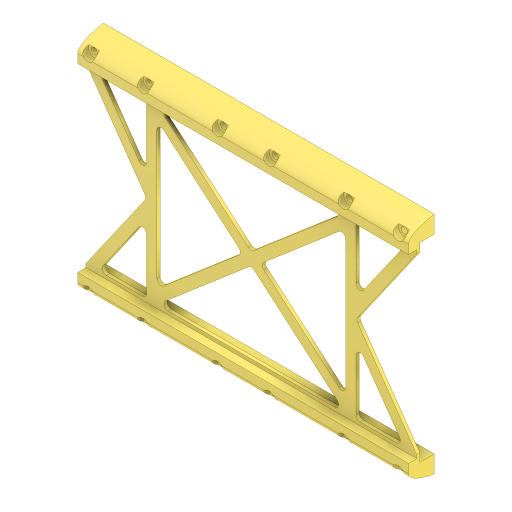
# Autodesk Inventor part: BodyStructure Centre V2
Saved by Autodesk Inventor 2023 (Build 270158000, 158)
## iProperties
Created: 2019-11-07
Part Number: BodyStructure Centre V2
Material: solidworks materials|ABS
Document SubType Name: Modeling
Designer: Jochen
Density: 1.02 g/cm^3
Appearance: 151,157,178
Sending System: SolidWorks 2017
Last Author: Felix
Last Saved: 2021-02-23
Author: Jochen
Autodesk Inventor part; units mm, degrees
ref_plane "YZ Plane" through (0, 0, 0) normal (1, 0, 0) x (0, 1, 0)
ref_plane "XZ Plane" through (0, 0, 0) normal (0, 1, 0) x (-1, 0, 0)
ref_plane "Work Plane1" through (0, 0, 30) normal (0, 0, 1) x (1, 0, 0)
sketch "Sketch1" plane through (0, 0, 30) normal (0, 0, 1) x (1, 0, 0)
  line L0 (-80, -56) -> (80, -56)
  line L1 (80, 56) -> (-80, 56)
  line L2 (80, 42) -> (80, 42)
  line L3 (0, -78.4) -> (0, 78.4) construction
  line L4 (-112, 0) -> (112, 0) construction
  line L5 (-50.6486, -42) -> (-50.6486, -8.7287)
  line L6 (-45.6486, 35.4185) -> (-45.6486, -35.4185)
  line L7 (-50.6486, -8.7287) -> (-73.9, -42)
  line L8 (-80, -42) -> (-50.6486, 0)
  line L9 (50.6486, -8.7287) -> (73.9, -42)
  line L10 (50.6486, -42) -> (50.6486, -8.7287)
  line L11 (45.6486, 35.4185) -> (45.6486, -35.4185)
  line L12 (80, -42) -> (50.6486, 0)
  line L13 (50.6486, 8.7287) -> (73.9, 42)
  line L14 (80, 42) -> (50.6486, 0)
  line L15 (50.6486, 0) -> (50.6486, 0)
  line L16 (50.6486, 8.7287) -> (50.6486, 42)
  line L17 (-50.6486, 0) -> (-50.6486, 0)
  line L18 (-80, 42) -> (-50.6486, 0)
  line L19 (-50.6486, 8.7287) -> (-73.9, 42)
  line L20 (-80, 42) -> (-80, 42)
  line L21 (-50.6486, 8.7287) -> (-50.6486, 42)
  line L22 (73.9, 42) -> (50.6486, 42)
  line L23 (-73.9, 42) -> (-50.6486, 42)
  line L24 (-45.6486, 42) -> (45.6486, 42)
  line L25 (-80, -42) -> (-80, -42)
  line L26 (-50.6486, -42) -> (-73.9, -42)
  line L27 (45.6486, -42) -> (-45.6486, -42)
  line L28 (80, -42) -> (80, -42)
  line L29 (73.9, -42) -> (50.6486, -42)
  line L30 (80, -56) -> (80, -42)
  line L31 (80, 42) -> (80, 56)
  line L32 (-80, 56) -> (-80, 42)
  line L33 (-80, -42) -> (-80, -56)
  line L34 (-48.1486, 56) -> (-48.1486, -56) construction
  line L35 (-45.6486, 42) -> (0, 2.927)
  line L36 (0, 2.927) -> (45.6486, 42)
  line L37 (45.6486, 35.4185) -> (4.2696, 0)
  line L38 (45.6486, -35.4185) -> (4.2696, 0)
  line L39 (0, -2.927) -> (45.6486, -42)
  line L40 (-4.2696, 0) -> (-45.6486, 35.4185)
  line L41 (-4.2696, 0) -> (-45.6486, -35.4185)
  line L42 (0, -2.927) -> (-45.6486, -42)
  point P0 (0, 0)
  point P1 (-2.5, 42)
  point P2 (2.5, 42)
  point P3 (2.5, -42)
  point P4 (-2.5, -42)
  point P5 (50.6486, 0)
  point P6 (-50.6486, 0)
  dimension "d2" = 5
  dimension "d3" = 0
  dimension "d4" = 160
  dimension "d5" = 14
  dimension "d7" = 112
  dimension "d101" = 5
  dimension "d107" = 5
  constraints: 82 end point, 17 parallel, 15 collinear, 15 perpendicular, 11 point on line, 9 horizontal, 2 vertical, 19 other
  measures "d2" distance between parallel lines of L6 L5
  measures "d3" distance of L8.start L25.end
  measures "d4" distance of L0.start L0.end
  measures "d5" distance of L25.end L0.start
  measures "d7" distance between parallel lines of L1 L0
  measures "d101" distance between parallel lines of L8 L7
  measures "d107" distance between parallel lines of L42 L41
extrude "Extrusion1" add sketch "Sketch1" along normal blind 20 and the other way blind 3.5
fillet "Fillet1" radius 2 22 edges at (-50.6486, -42, 38.25) (-50.6486, -8.7287, 38.25) (-73.9, -42, 38.25) (-73.9, 42, 38.25) (-50.6486, 42, 38.25) (-50.6486, 8.7287, 38.25) (50.6486, -8.7287, 38.25) (50.6486, -42, 38.25) (50.6486, 42, 38.25) (50.6486, 8.7287, 38.25) (73.9, 42, 38.25) (73.9, -42, 38.25) (-45.6486, 35.4185, 38.25) (0, -2.927, 38.25) (4.2696, 0, 38.25) (0, 2.927, 38.25) (-4.2696, 0, 38.25) (-45.6486, -35.4185, 38.25) (45.6486, -35.4185, 38.25) (45.6486, 35.4185, 38.25) (50.6486, 0, 38.25) (-50.6486, 0, 38.25)
fillet "Fillet1" radius 2 4 edges at (-45.6486, 42, 38.25) (-45.6486, -42, 38.25) (45.6486, -42, 38.25) (45.6486, 42, 38.25)
sketch "Sketch12" plane through (80, -56, 30) normal (1, 0, 0) x (0, 0, -1)
  line L0 (-4.5, 0) -> (-17, 0)
  line L1 (-17, 112) -> (-1.5, 112)
  line L2 (-17, 99.75) -> (-17, 104)
  line L3 (-17, 0) -> (-17, 8)
  line L4 (-17, 8) -> (45, 8) construction
  line L5 (-17, 104) -> (45, 104) construction
  ellipse E0 centre (14, 8) end of major axis (-17, 8) minor radius 8 (-17, 8) -> (45, 8) ccw
  ellipse E1 centre (14, 104) end of major axis (-17, 104) minor radius 8 (45, 104) -> (-17, 104) ccw
  line L6 (-17, 8) -> (-17, 0)
  line L7 (-17, 0) -> (14, 0)
  line L8 (-17, 112) -> (14, 112)
  line L9 (-17, 12.25) -> (-13, 12.25)
  line L10 (-13, 12.25) -> (-13, 14)
  line L11 (-13, 98) -> (-13, 99.75)
  line L12 (-13, 99.75) -> (-17, 99.75)
  line L13 (-17, 104) -> (-17, 99.75)
  line L14 (-17, 99.75) -> (-13, 99.75)
  line L15 (-13, 99.75) -> (-13, 98)
  line L16 (30, -22.4) -> (30, 134.4) construction
  line L17 (54.4, 56) -> (-32.4, 56) construction
  line L18 (-17, 8) -> (-17, 12.25)
  line L19 (-17, 104) -> (-17, 112)
  line L20 (-13, 98) -> (-13, 14)
  line L21 (-11.5, 14) -> (-11.5, 98)
  line L22 (-4.5, 10) -> (-11.5, 10)
  line L23 (-11.5, 10) -> (-11.5, 14)
  line L24 (-4.5, 102) -> (-11.5, 102)
  line L25 (-11.5, 102) -> (-11.5, 98)
  line L26 (-13, 14) -> (-13, 14)
  line L27 (-4.5, 110.4193) -> (-4.5, 102)
  line L28 (-4.5, 10) -> (-4.5, 0)
  line L29 (0, 10) -> (0, 8)
  line L30 (0, 14) -> (0, 54.8543) projected
  point P0 (30, 56)
  point P1 (0, 13)
  point P2 (-13, 14)
  point P3 (-8, 110.3213)
  point P4 (-11.5, 14)
  point P5 (-4.5, 1.5807)
  dimension "d139" = 62
  dimension "d140" = 8
  dimension "d148" = 96
  dimension "d149" = 1.75
  dimension "d150" = 4
  dimension "d152" = 4.25
  dimension "d154" = 1.5
  dimension "d157" = 12.5
  dimension "d159" = 92
  dimension "d160" = 17
  constraints: 56 end point, 11 perpendicular, 10 horizontal, 4 collinear, 4 point on line, 3 equal length, 3 midpoint, 3 vertical, 14 other
  measures "d139" distance of L4.end L3.end
  measures "d140" distance between parallel lines of L4 L0
  measures "d148" distance between parallel lines of L4 L5
  measures "d149" distance of L9.end L10.end
  measures "d150" distance of L9.start L9.end
  measures "d152" distance from line of L9 L3.end
  measures "d154" distance between parallel lines of L20 L21
  measures "d157" distance between parallel lines of L3 L28
  measures "d159" distance between parallel lines of L24 L22
  measures "d160" distance between parallel lines of L30 L3
extrude "Extrusion16" cut sketch "Sketch12" against normal through all contours E0 L18 L9 L10 L20 L11 L12 L2 E1 L27 L24 L25 L21 L23 L22 L28 keep common part
sketch "Sketch9" plane through (45, -54.8115, 43) normal (0, 0, -1) x (-1, 0, 0)
  circle A0 centre (-30, 104.8115) radius 1.5
  circle A1 centre (32.5, 104.8115) radius 1.5
  circle A2 centre (-3.5, 104.8115) radius 1.5
  circle A3 centre (57.5, 104.8115) radius 1.5
  circle A4 centre (93.5, 104.8115) radius 1.5
  circle A5 centre (120, 104.8115) radius 1.5
  circle A6 centre (120, 4.8115) radius 1.5
  circle A7 centre (93.5, 4.8115) radius 1.5
  circle A8 centre (57.5, 4.8115) radius 1.5
  circle A9 centre (-3.5, 4.8115) radius 1.5
  circle A10 centre (32.5, 4.8115) radius 1.5
  circle A11 centre (-30, 4.8115) radius 1.5
  line L0 (-30, 104.8115) -> (120, 104.8115) construction
  line L1 (120, 104.8115) -> (120, 4.8115) construction
  line L2 (120, 4.8115) -> (-30, 4.8115) construction
  line L3 (-30, 4.8115) -> (-30, 104.8115) construction
  line L4 (157, 54.8115) -> (-67, 54.8115) construction
  line L5 (45, -22.0635) -> (45, 131.9365) construction
  line L6 (32.5, 104.8115) -> (32.5, 4.8115) construction
  line L7 (-3.5, 4.8115) -> (-3.5, 104.8115) construction
  line L8 (93.5, 104.8115) -> (93.5, 4.8115) construction
  line L9 (57.5, 104.8115) -> (57.5, 4.8115) construction
  circle A12 centre (-30, 4.8115) radius 2.9
  circle A13 centre (-3.5, 4.8115) radius 2.9
  circle A14 centre (32.5, 4.8115) radius 2.9
  circle A15 centre (57.5, 4.8115) radius 2.9
  circle A16 centre (93.5, 4.8115) radius 2.9
  circle A17 centre (120, 4.8115) radius 2.9
  circle A18 centre (120, 104.8115) radius 2.9
  circle A19 centre (93.5, 104.8115) radius 2.9
  circle A20 centre (57.5, 104.8115) radius 2.9
  circle A21 centre (32.5, 104.8115) radius 2.9
  circle A22 centre (-3.5, 104.8115) radius 2.9
  circle A23 centre (-30, 104.8115) radius 2.9
  line L10 (97.7, 1.4365) -> (97.7, -0.0635)
  line L11 (-7.7, -0.0635) -> (-7.7, 1.4365)
  line L12 (125, 106.7422) -> (-35, 106.7422) projected
  line L13 (-35, 106.7422) -> (-35, 98.5615) projected
  line L14 (125, 98.5615) -> (125, 106.7422) projected
  line L15 (125, 11.0615) -> (125, 12.8115) projected
  line L16 (125, 11.0615) -> (-35, 11.0615) projected
  line L17 (-35, 11.0615) -> (-35, 2.8808) projected
  line L18 (-35, 2.8808) -> (125, 2.8808) projected
  line L19 (125, 2.8808) -> (125, 11.0615) projected
  line L20 (-35, 12.8115) -> (-35, 11.0615) projected
  line L21 (-6.4493, 53.6658) -> (-35, 12.8115) projected
  arc A24 (-6.4493, 53.6658) -> (-6.4493, 55.9571) centre (-8.0886, 54.8115) ccw projected
  line L22 (-35, 96.8115) -> (-6.4493, 55.9571) projected
  line L23 (-35, 98.5615) -> (-35, 96.8115) projected
  line L24 (-35, 98.5615) -> (125, 98.5615) projected
  line L25 (125, 12.8115) -> (96.4493, 53.6658) projected
  arc A25 (96.4493, 55.9571) -> (96.4493, 53.6658) centre (98.0886, 54.8115) ccw projected
  line L26 (96.4493, 55.9571) -> (125, 96.8115) projected
  line L27 (125, 96.8115) -> (125, 98.5615) projected
  arc A26 (46.3005, 50.7713) -> (43.6995, 50.7713) centre (45, 49.2519) ccw projected
  line L28 (46.3005, 50.7713) -> (86.537, 16.3309) projected
  arc A27 (85.2364, 12.8115) -> (86.537, 16.3309) centre (85.2364, 14.8115) ccw projected
  line L29 (85.2364, 12.8115) -> (4.7636, 12.8115) projected
  arc A28 (3.463, 16.3309) -> (4.7636, 12.8115) centre (4.7636, 14.8115) ccw projected
  line L30 (3.463, 16.3309) -> (43.6995, 50.7713) projected
  arc A29 (38.9553, 53.2921) -> (38.9553, 56.3309) centre (37.6548, 54.8115) ccw projected
  line L31 (38.9553, 53.2921) -> (2.6519, 22.2181) projected
  arc A30 (-0.6486, 23.7375) -> (2.6519, 22.2181) centre (1.3514, 23.7375) ccw projected
  line L32 (-0.6486, 23.7375) -> (-0.6486, 85.8855) projected
  arc A31 (2.6519, 87.4049) -> (-0.6486, 85.8855) centre (1.3514, 85.8855) ccw projected
  line L33 (2.6519, 87.4049) -> (38.9553, 56.3309) projected
  arc A32 (-5.6486, 39.7295) -> (-9.288, 40.8751) centre (-7.6486, 39.7295) ccw projected
  line L34 (-5.6486, 39.7295) -> (-5.6486, 14.8115) projected
  arc A33 (-7.6486, 12.8115) -> (-5.6486, 14.8115) centre (-7.6486, 14.8115) ccw projected
  line L35 (-7.6486, 12.8115) -> (-25.0624, 12.8115) projected
  arc A34 (-26.7017, 15.9571) -> (-25.0624, 12.8115) centre (-25.0624, 14.8115) ccw projected
  line L36 (-26.7017, 15.9571) -> (-9.288, 40.8751) projected
  arc A35 (-5.6486, 94.8115) -> (-7.6486, 96.8115) centre (-7.6486, 94.8115) ccw projected
  line L37 (-5.6486, 94.8115) -> (-5.6486, 69.8935) projected
  arc A36 (-9.288, 68.7479) -> (-5.6486, 69.8935) centre (-7.6486, 69.8935) ccw projected
  line L38 (-9.288, 68.7479) -> (-26.7017, 93.6658) projected
  arc A37 (-25.0624, 96.8115) -> (-26.7017, 93.6658) centre (-25.0624, 94.8115) ccw projected
  line L39 (-25.0624, 96.8115) -> (-7.6486, 96.8115) projected
  arc A38 (95.6486, 14.8115) -> (97.6486, 12.8115) centre (97.6486, 14.8115) ccw projected
  line L40 (95.6486, 14.8115) -> (95.6486, 39.7295) projected
  arc A39 (99.288, 40.8751) -> (95.6486, 39.7295) centre (97.6486, 39.7295) ccw projected
  line L41 (99.288, 40.8751) -> (116.7017, 15.9571) projected
  arc A40 (115.0624, 12.8115) -> (116.7017, 15.9571) centre (115.0624, 14.8115) ccw projected
  line L42 (115.0624, 12.8115) -> (97.6486, 12.8115) projected
  arc A41 (4.7636, 96.8115) -> (3.463, 93.2921) centre (4.7636, 94.8115) ccw projected
  line L43 (4.7636, 96.8115) -> (85.2364, 96.8115) projected
  arc A42 (86.537, 93.2921) -> (85.2364, 96.8115) centre (85.2364, 94.8115) ccw projected
  line L44 (86.537, 93.2921) -> (46.3005, 58.8516) projected
  arc A43 (43.6995, 58.8516) -> (46.3005, 58.8516) centre (45, 60.371) ccw projected
  line L45 (43.6995, 58.8516) -> (3.463, 93.2921) projected
  arc A44 (87.3481, 22.2181) -> (90.6486, 23.7375) centre (88.6486, 23.7375) ccw projected
  line L46 (87.3481, 22.2181) -> (51.0447, 53.2921) projected
  arc A45 (51.0447, 56.3309) -> (51.0447, 53.2921) centre (52.3452, 54.8115) ccw projected
  line L47 (51.0447, 56.3309) -> (87.3481, 87.4049) projected
  arc A46 (90.6486, 85.8855) -> (87.3481, 87.4049) centre (88.6486, 85.8855) ccw projected
  line L48 (90.6486, 85.8855) -> (90.6486, 23.7375) projected
  arc A47 (95.6486, 69.8935) -> (99.288, 68.7479) centre (97.6486, 69.8935) ccw projected
  line L49 (95.6486, 69.8935) -> (95.6486, 94.8115) projected
  arc A48 (97.6486, 96.8115) -> (95.6486, 94.8115) centre (97.6486, 94.8115) ccw projected
  line L50 (97.6486, 96.8115) -> (115.0624, 96.8115) projected
  arc A49 (116.7017, 93.6658) -> (115.0624, 96.8115) centre (115.0624, 94.8115) ccw projected
  line L51 (116.7017, 93.6658) -> (99.288, 68.7479) projected
  point P0 (45, 54.8115)
  point P1 (42.5, 12.9365)
  point P2 (-6, 80.6486)
  point P3 (-6, 19.2244)
  point P4 (-6, 14.9365)
  point P5 (47.5, 86.9365)
  point P6 (42.5, 76.9365)
  point P7 (42.5, 22.9365)
  point P8 (47.5, 76.9365)
  point P9 (47.5, 22.9365)
  point P10 (-6, 36.0374)
  point P11 (98.4175, 46.8521)
  point P12 (45, 52.0098)
  point P13 (45, 57.8631)
  point P14 (-5.649, 54.9365)
  point P15 (95.649, 54.9365)
  point P16 (0, 109.9365)
  point P17 (36, -0.0635)
  point P18 (29, -0.0635)
  point P19 (0, -0.0635)
  point P20 (1, 109.9365)
  point P21 (28, 109.9365)
  point P22 (37, 109.9365)
  point P23 (62, 109.9365)
  point P24 (89, 109.9365)
  point P25 (98, 109.9365)
  point P26 (89, -0.0635)
  point P27 (62, -0.0635)
  point P28 (53, -0.0635)
  point P29 (37, -0.0635)
  point P30 (28, -0.0635)
  point P31 (1, -0.0635)
  point P32 (-8, -0.0635)
  point P33 (0, 101.8115)
  point P34 (90, 101.8115)
  point P35 (90, 8.0615)
  point P36 (0, 8.0615)
  point P37 (36.5, -0.0635)
  point P38 (16.5, 109.9365)
  dimension "d61" = 3
  dimension "d63" = 100
  dimension "d64" = 75
  dimension "d65" = 48.5
  dimension "d66" = 12.5
  dimension "d69" = 5.8
  constraints: 24 centre point, 22 equal radius, 20 end point, 15 coincident, 8 point on line, 3 parallel, 3 vertical, 1 horizontal, 1 perpendicular, 5 other
  measures "d61" diameter of A0
  measures "d63" distance of L2.end L0.start
  measures "d64" distance from line of A11.centre L5
  measures "d65" distance from line of L7.start L5
  measures "d66" distance from line of L6.end L5
  measures "d69" diameter of A12
extrude "Extrusion8" cut sketch "Sketch9" along normal through all both and the other way through all contours A0 | A1 | A2 | A3 | A4 | A5 | A6 | A7 | A8 | A9 | A10 | A11
extrude "Extrusion9" cut sketch "Sketch9" along normal blind 6 from surface at -7 contours A0 | A1 | A2 | A3 | A4 | A5 | A6 | A7 | A8 | A9 | A10 | A11 | A12 L18 | L18 A12 | L18 A13 | A13 L18 | L18 A14 | A14 L18 | L18 A17 | A17 L18 | L18 A15 | A15 L18 | L18 A16 | A16 L18 | L12 A23 | A23 L12 | L12 A18 | A18 L12 | L12 A22 | A22 L12 | L12 A19 | A19 L12 | L12 A21 | A21 L12 | L12 A20 | A20 L12
fillet "Fillet6" [suppressed]
equation "\"d2\" = d1"
equation "\"d1\" = 5"
body "Solid1"
body "Solid2"
